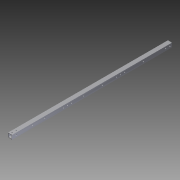
# Autodesk Inventor part: towertallbackthing
Saved by Autodesk Inventor 2011 SP1 (Build 150282100, 282)
## iProperties
Created: 2012-01-18
Part Number: towertallbackthing
Document SubType Name: Modeling
Designer: Christopher
Density: 1 g/cm^3
Author: Christopher
Autodesk Inventor part; units mm, degrees
ref_plane "YZ Plane" through (0, 0, 0) normal (1, 0, 0) x (0, 1, 0)
ref_plane "XZ Plane" through (0, 0, 0) normal (0, 1, 0) x (-1, 0, 0)
ref_plane "XY Plane" through (0, 0, 0) normal (0, 0, 1) x (1, 0, 0)
sketch "Sketch1" plane through (0, 0, 0) normal (0, 0, 1) x (1, 0, 0)
  line L0 (0, 0) -> (25.4, 0)
  line L1 (25.4, 0) -> (25.4, 25.4)
  line L2 (25.4, 25.4) -> (0, 25.4)
  line L3 (0, 25.4) -> (0, 0)
  line L4 (3.175, 3.175) -> (22.225, 3.175)
  line L5 (22.225, 3.175) -> (22.225, 22.225)
  line L6 (22.225, 22.225) -> (3.175, 22.225)
  line L7 (3.175, 22.225) -> (3.175, 3.175)
  dimension "d0" = 25.4
  dimension "d1" = 25.4
  dimension "d2" = 3.175
  constraints: 16 end point, 4 parallel, 2 perpendicular, 1 horizontal, 3 other
  measures "d0" distance of L1.end L2.end
  measures "d1" distance of L0.end L1.end
  measures "d2" distance between parallel lines of L3 L7
extrude "Extrusion1" add sketch "Sketch1" against normal blind 990.6
sketch "Sketch2" plane through (0, 0, -990.6) normal (-1, 0, 0) x (0, 0, 1)
  line L0 (990.6, 25.4) -> (990.6, 0) projected
  line L1 (990.6, 0) -> (0, 0) projected
  line L2 (0, 25.4) -> (0, 0) projected
  line L3 (990.6, 25.4) -> (0, 25.4) projected
  point P0 (965.2, 12.7)
  point P1 (787.4, 12.7)
  point P2 (431.8, 12.7)
  point P3 (76.2, 12.7)
  point P4 (673.1, 12.7)
  point P5 (647.7, 12.7)
  point P6 (622.3, 12.7)
  point P7 (342.9, 12.7)
  point P8 (317.5, 12.7)
  point P9 (292.1, 12.7)
  point P10 (787.4, 12.7)
  point P11 (546.1, 12.7)
  point P12 (177.8, 12.7)
  point P13 (863.6, 12.7)
  point P14 (12.7, 12.7)
  point P15 (38.1, 12.7)
  dimension "d33" = 317.5
  dimension "d34" = 25.4
  dimension "d35" = 25.4
  dimension "d36" = 279.4
  dimension "d37" = 25.4
  dimension "d38" = 25.4
  dimension "d46" = 114.3
  dimension "d47" = 76.2
  dimension "d48" = 12.7
  dimension "d49" = 114.3
  dimension "d50" = 127
  dimension "d51" = 12.7
  dimension "d52" = 25.4
  dimension "d53" = 12.7
  constraints: 1 coincident
  measures "d33" distance from line of point (673.1, 12.7) L0
  measures "d34" distance of point (647.7, 12.7) point (673.1, 12.7)
  measures "d35" distance of point (622.3, 12.7) point (647.7, 12.7)
  measures "d36" distance of point (342.9, 12.7) point (622.3, 12.7)
  measures "d37" distance of point (317.5, 12.7) point (342.9, 12.7)
  measures "d38" distance of point (292.1, 12.7) point (317.5, 12.7)
  measures "d46" distance of point (673.1, 12.7) point (787.4, 12.7)
  measures "d47" distance of point (546.1, 12.7) point (622.3, 12.7)
  measures "d48" distance from line of L1 point (177.8, 12.7)
  measures "d49" distance of point (292.1, 12.7) point (177.8, 12.7)
  measures "d50" distance from line of L0 point (863.6, 12.7)
  measures "d51" distance from line of L2 point (12.7, 12.7)
  measures "d52" distance of point (38.1, 12.7) point (12.7, 12.7)
  measures "d53" distance from line of L3 point (38.1, 12.7)
sketch "Sketch3" plane through (0, 0, 0) normal (0, -1, 0) x (1, 0, 0)
  line L0 (0, 0) -> (25.4, 0) projected
  point P0 (12.7, -12.7)
  point P1 (12.7, -38.1)
  dimension "d24" = 25.4
  dimension "d25" = 12.7
  measures "d24" distance of point (12.7, -38.1) point (12.7, -12.7)
  measures "d25" distance from line of point (12.7, -12.7) L0
hole "Hole3" at (12.7, 0, -12.7) at (12.7, 0, -38.1) direction (0, 1, 0) diameter 6.35 depth 25.4 tip angle 118
hole "Hole4" at (0, 12.7, -317.5) at (0, 12.7, -342.9) at (0, 12.7, -368.3) at (0, 12.7, -647.7) at (0, 12.7, -673.1) at (0, 12.7, -698.5) at (0, 12.7, -444.5) at (0, 12.7, -812.8) at (0, 12.7, -127) direction (1, 0, 0) diameter 6.35 depth 25.4 tip angle 118
hole "Hole5" at (0, 12.7, -25.4) at (0, 12.7, -203.2) at (0, 12.7, -558.8) at (0, 12.7, -977.9) at (0, 12.7, -952.5) direction (1, 0, 0) diameter 6.35 depth 25.4 tip angle 118
body "Solid1"
